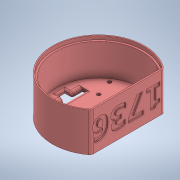
# Autodesk Inventor part: camHolderBottom
Saved by Autodesk Inventor 2020 (Build 240168000, 168)
## iProperties
Created: 2020-02-08
Part Number: camHolderBottom
Material: Generic
Document SubType Name: Modeling
Designer: Chris Gerth
Density: 1 g/cm^3
Appearance: Default(1)
Author: Chris Gerth
Autodesk Inventor part; units mm, degrees
ref_plane "YZ Plane" through (0, 0, 0) normal (1, 0, 0) x (0, 1, 0)
ref_plane "XZ Plane" through (0, 0, 0) normal (0, 1, 0) x (-1, 0, 0)
ref_plane "XY Plane" through (0, 0, 0) normal (0, 0, 1) x (1, 0, 0)
sketch "Sketch1" plane through (0, 0, 0) normal (0, 1, 0) x (-1, 0, 0)
  arc A0 (-25.4, -31.7246) -> (-25.4, 31.7246) centre (0, 0) ccw
  line L0 (-25.4, 31.7246) -> (-25.4, -31.7246)
  dimension "d0" = 81.28
  dimension "d31" = 25.4
  constraints: 2 end point, 2 point on circle, 1 centre point, 1 coincident, 1 vertical
  measures "d0" diameter of A0
  measures "d31" distance from line of L0 point (0, 0)
extrude "Extrusion1" add sketch "Sketch1" along normal blind 3.175
sketch "Sketch2" plane through (0, 3.175, 0) normal (0, 1, 0) x (0, 0, 1)
  arc A0 (-31.7246, 25.4) -> (31.7246, 25.4) centre (0, 0) ccw
  arc A1 (-30.9461, 22.225) -> (30.9461, 22.225) centre (0, 0) ccw
  arc A2 (-31.7246, 25.4) -> (31.7246, 25.4) centre (0, 0) ccw projected
  line L0 (31.7246, 25.4) -> (-31.7246, 25.4)
  line L1 (30.9461, 22.225) -> (-30.9461, 22.225)
  dimension "d3" = 76.2
  dimension "d32" = 3.175
  constraints: 4 end point, 4 point on circle, 2 centre point, 2 coincident, 2 horizontal
  measures "d3" diameter of A1
  measures "d32" distance between parallel lines of L0 L1
extrude "Extrusion2" add sketch "Sketch2" along normal blind 27.94
sketch "Sketch3" plane through (0, 31.115, 0) normal (0, 1, 0) x (0, 0, 1)
  arc A0 (-31.7246, 25.4) -> (31.7246, 25.4) centre (0, 0) ccw
  arc A1 (-31.7246, 25.4) -> (31.7246, 25.4) centre (0, 0) ccw
  arc A2 (-31.5893, 24.13) -> (31.5893, 24.13) centre (0, 0) ccw
  arc A3 (-31.7246, 25.4) -> (31.7246, 25.4) centre (0, 0) ccw projected
  line L0 (31.7246, 25.4) -> (-31.7246, 25.4)
  line L1 (31.5893, 24.13) -> (-31.5893, 24.13)
  dimension "d6" = 79.502
  dimension "d33" = 1.27
  constraints: 6 point on circle, 4 end point, 3 centre point, 3 coincident, 2 horizontal
  measures "d6" diameter of A2
  measures "d33" distance between parallel lines of L0 L1
extrude "Extrusion3" add sketch "Sketch3" along normal blind 3.175
sketch "Sketch4" plane through (0, 3.175, 0) normal (0, 1, 0) x (0, 0, 1)
  line L0 (-14.4, 14.4) -> (14.4, 14.4)
  line L1 (14.4, 14.4) -> (14.4, -14.4)
  line L2 (14.4, -14.4) -> (-14.4, -14.4)
  line L3 (-14.4, -14.4) -> (-14.4, 14.4)
  line L4 (-14.4, 14.4) -> (14.4, -14.4) construction
  line L5 (14.4, 14.4) -> (-14.4, -14.4) construction
  circle A0 centre (-14.4, 14.4) radius 1.55
  circle A1 centre (14.4, 14.4) radius 1.55
  circle A2 centre (-14.4, -14.4) radius 1.55
  circle A3 centre (14.4, -14.4) radius 1.55
  point P0 (0, 0)
  dimension "d9" = 28.8
  dimension "d10" = 28.8
  dimension "d11" = 3.1
  dimension "d12" = 3.1
  dimension "d13" = 3.1
  dimension "d14" = 3.1
  constraints: 12 end point, 4 centre point, 4 coincident, 2 midpoint, 2 parallel, 1 horizontal, 1 perpendicular
  measures "d9" distance of L1.end L2.end
  measures "d10" distance of L2.end L0.start
  measures "d11" diameter of A0
  measures "d12" diameter of A1
  measures "d13" diameter of A2
  measures "d14" diameter of A3
extrude "Extrusion4" cut sketch "Sketch4" against normal up to surface (3.175 mm away) contours L3 A0 L0 | L0 A0 L3 | A1 L1 L0 | L0 L1 A1 | A2 L2 L3 | L3 L2 A2 | A3 L2 L1 | L1 L2 A3
sketch "Sketch5" plane through (0, 3.175, 0) normal (0, 1, 0) x (0, 0, 1)
  line L0 (12.7, -23.7415) -> (-12.7, -23.7415)
  line L1 (-12.7, -23.7415) -> (-12.7, -26.9165)
  line L2 (-12.7, -26.9165) -> (12.7, -26.9165)
  line L3 (12.7, -26.9165) -> (12.7, -23.7415)
  line L4 (12.7, -23.7415) -> (-12.7, -26.9165) construction
  line L5 (-12.7, -23.7415) -> (12.7, -26.9165) construction
  line L6 (3.5906, -33.2771) -> (3.5906, -25.329)
  line L7 (3.5906, -25.329) -> (-3.5906, -25.329)
  line L8 (-3.5906, -25.329) -> (-3.5906, -33.2771)
  line L9 (-3.5906, -33.2771) -> (3.5906, -33.2771)
  line L10 (3.5906, -33.2771) -> (-3.5906, -25.329) construction
  line L11 (3.5906, -25.329) -> (-3.5906, -33.2771) construction
  point P0 (0, 0)
  point P1 (0, -25.329)
  point P2 (0, -29.303)
  point P3 (3.5906, -26.9165)
  point P4 (-3.5906, -26.9165)
  dimension "d17" = 25.4
  dimension "d18" = 3.175
  constraints: 24 end point, 4 midpoint, 4 parallel, 2 perpendicular, 1 vertical
  measures "d17" distance of L0.start L0.end
  measures "d18" distance of L1.end L0.end
extrude "Extrusion5" cut sketch "Sketch5" against normal up to surface (3.175 mm away)
sketch "Sketch6" plane through (0, 3.175, 0) normal (0, 1, 0) x (0, 0, 1)
  line L0 (28.575, 19.05) -> (28.575, -19.05)
  line L1 (28.575, -19.05) -> (-28.575, -19.05)
  line L2 (-28.575, -19.05) -> (-28.575, 19.05)
  line L3 (-28.575, 19.05) -> (28.575, 19.05)
  line L4 (28.575, 19.05) -> (-28.575, -19.05) construction
  line L5 (28.575, -19.05) -> (-28.575, 19.05) construction
  circle A0 centre (-28.575, -19.05) radius 1.55
  circle A1 centre (-28.575, 19.05) radius 1.55
  circle A2 centre (28.575, 19.05) radius 1.55
  circle A3 centre (28.575, -19.05) radius 1.55
  point P0 (0, 0)
  dimension "d21" = 38.1
  dimension "d22" = 57.15
  dimension "d23" = 3.1
  dimension "d24" = 3.1
  dimension "d25" = 3.1
  dimension "d26" = 3.1
  constraints: 12 end point, 4 centre point, 4 coincident, 2 parallel, 1 perpendicular
  measures "d21" distance of L1.end L2.end
  measures "d22" distance of L0.end L1.end
  measures "d23" diameter of A0
  measures "d24" diameter of A1
  measures "d25" diameter of A2
  measures "d26" diameter of A3
extrude "Extrusion6" cut sketch "Sketch6" against normal blind 3.175 contours L3 A2 L0 | L0 A2 L3 | A3 L1 L0 | L0 L1 A3 | A1 L2 L3 | L3 L2 A1 | A0 L2 L1 | L1 L2 A0
sketch "Sketch7" plane through (25.4, 0, 31.7246) normal (1, 0, 0) x (0, 0, -1)
  line L0 (62.4595, 7.7021) -> (-13.7817, 7.7021) construction
  line L1 (-13.7817, 7.7021) -> (-13.7817, 34.1724) construction
  line L2 (-13.7817, 34.1724) -> (62.4595, 34.1724) construction
  line L3 (62.4595, 34.1724) -> (62.4595, 7.7021) construction
  line L4 (48.3825, 25.8567) -> (60.1253, 25.8567)
  line L5 (60.1253, 25.8567) -> (60.1253, 22.7589)
  line L6 (60.1253, 22.7589) -> (56.3791, 22.7589)
  line L7 (56.3791, 22.7589) -> (56.3791, 13.3502)
  line L8 (56.3791, 13.3502) -> (60.1253, 13.3502)
  line L9 (60.1253, 13.3502) -> (60.1253, 10.4541)
  spline S0 degree 2 poles (60.1253, 10.4541) (59.304, 10.4541) (57.6759, 10.2379) (57.186, 10.0074) knots 0 0 0 1 2 2 2
  spline S1 degree 2 poles (57.186, 10.0074) (56.6241, 9.7192) (55.9901, 8.7539) (55.9325, 8.0335) knots 0 0 0 1 2 2 2
  line L10 (55.9325, 8.0335) -> (52.0422, 8.0335)
  line L11 (52.0422, 8.0335) -> (52.0422, 22.7589)
  line L12 (52.0422, 22.7589) -> (48.3825, 22.7589)
  line L13 (48.3825, 22.7589) -> (48.3825, 25.8567)
  line L14 (32.4035, 11.6067) -> (39.9967, 25.8567)
  line L15 (39.9967, 25.8567) -> (44.9532, 25.8567)
  line L16 (44.9532, 25.8567) -> (37.0142, 11.4338)
  line L17 (37.0142, 11.4338) -> (45.4864, 11.4338)
  line L18 (45.4864, 11.4338) -> (45.4864, 8.0767)
  line L19 (45.4864, 8.0767) -> (32.4035, 8.0767)
  line L20 (32.4035, 8.0767) -> (32.4035, 11.6067)
  spline S2 degree 2 poles (16.8856, 20.4679) (16.8856, 21.7791) (17.851, 23.926) (18.7875, 24.6752) knots 0 0 0 1 2 2 2
  spline S3 degree 2 poles (18.7875, 24.6752) (19.7241, 25.4244) (22.2744, 26.2313) (24.1043, 26.2313) knots 0 0 0 1 2 2 2
  spline S4 degree 2 poles (24.1043, 26.2313) (26.1791, 26.2313) (29.1472, 25.5397) (30.0837, 25.1074) knots 0 0 0 1 2 2 2
  line L21 (30.0837, 25.1074) -> (30.0837, 21.246)
  line L22 (30.0837, 21.246) -> (29.6515, 21.246)
  spline S5 degree 2 poles (29.6515, 21.246) (28.6717, 21.8655) (26.035, 22.7877) (24.9399, 22.7877) knots 0 0 0 1 2 2 2
  spline S6 degree 2 poles (24.9399, 22.7877) (24.2916, 22.7877) (22.7787, 22.5572) (22.26, 22.1825) knots 0 0 0 1 2 2 2
  spline S7 degree 2 poles (22.26, 22.1825) (21.8565, 21.88) (21.3666, 21.001) (21.3666, 20.2086) knots 0 0 0 1 2 2 2
  spline S8 degree 2 poles (21.3666, 20.2086) (21.3666, 19.4161) (22.0583, 18.566) (22.6346, 18.3643) knots 0 0 0 1 2 2 2
  spline S9 degree 2 poles (22.6346, 18.3643) (23.2109, 18.1626) (24.8103, 18.1194) (25.4298, 18.1194) knots 0 0 0 1 2 2 2
  line L23 (25.4298, 18.1194) -> (26.1935, 18.1194)
  line L24 (26.1935, 18.1194) -> (26.1935, 14.9927)
  line L25 (26.1935, 14.9927) -> (25.4875, 14.9927)
  spline S10 degree 2 poles (25.4875, 14.9927) (24.6806, 14.9927) (23.3118, 14.8486) (22.8363, 14.6325) knots 0 0 0 1 2 2 2
  spline S11 degree 2 poles (22.8363, 14.6325) (22.3608, 14.402) (21.8277, 13.5951) (21.8277, 12.9035) knots 0 0 0 1 2 2 2
  spline S12 degree 2 poles (21.8277, 12.9035) (21.8277, 12.356) (22.332, 11.6788) (22.6922, 11.4915) knots 0 0 0 1 2 2 2
  spline S13 degree 2 poles (22.6922, 11.4915) (23.1245, 11.2754) (24.2772, 11.1313) (24.6806, 11.1313) knots 0 0 0 1 2 2 2
  spline S14 degree 2 poles (24.6806, 11.1313) (25.329, 11.1313) (26.6978, 11.4338) (27.3317, 11.6788) knots 0 0 0 1 2 2 2
  spline S15 degree 2 poles (27.3317, 11.6788) (27.836, 11.8661) (28.9311, 12.4713) (29.1904, 12.6297) knots 0 0 0 1 2 2 2
  line L26 (29.1904, 12.6297) -> (29.565, 12.6297)
  line L27 (29.565, 12.6297) -> (29.565, 8.8259)
  spline S16 degree 2 poles (29.565, 8.8259) (28.6429, 8.4369) (25.5307, 7.7021) (23.9025, 7.7021) knots 0 0 0 1 2 2 2
  spline S17 degree 2 poles (23.9025, 7.7021) (22.3176, 7.7021) (19.9834, 8.2496) (19.1622, 8.7827) knots 0 0 0 1 2 2 2
  spline S18 degree 2 poles (19.1622, 8.7827) (18.2544, 9.3446) (17.3467, 11.0736) (17.3467, 12.1543) knots 0 0 0 1 2 2 2
  spline S19 degree 2 poles (17.3467, 12.1543) (17.3467, 13.6816) (19.1045, 15.9581) (20.5454, 16.2895) knots 0 0 0 1 2 2 2
  line L28 (20.5454, 16.2895) -> (20.5454, 16.4624)
  spline S20 degree 2 poles (20.5454, 16.4624) (19.9114, 16.5488) (18.7011, 17.0099) (18.1248, 17.5286) knots 0 0 0 1 2 2 2
  spline S21 degree 2 poles (18.1248, 17.5286) (17.5916, 17.9897) (16.8856, 19.4593) (16.8856, 20.4679) knots 0 0 0 1 2 2 2
  spline S22 degree 2 poles (0.9643, 19.8051) (0.9643, 22.6148) (4.5232, 26.2313) (7.6354, 26.2313) knots 0 0 0 1 2 2 2
  spline S23 degree 2 poles (7.6354, 26.2313) (9.1915, 26.2313) (11.6266, 25.338) (12.4766, 24.4591) knots 0 0 0 1 2 2 2
  spline S24 degree 2 poles (12.4766, 24.4591) (13.4852, 23.4361) (14.5659, 20.1942) (14.5659, 17.932) knots 0 0 0 1 2 2 2
  spline S25 degree 2 poles (14.5659, 17.932) (14.5659, 15.5979) (13.5573, 11.967) (12.419, 10.5693) knots 0 0 0 1 2 2 2
  spline S26 degree 2 poles (12.419, 10.5693) (11.3384, 9.2438) (7.8227, 7.7453) (5.4165, 7.7453) knots 0 0 0 1 2 2 2
  spline S27 degree 2 poles (5.4165, 7.7453) (4.5376, 7.7453) (2.7798, 7.9758) (2.4628, 8.0479) knots 0 0 0 1 2 2 2
  line L29 (2.4628, 8.0479) -> (2.4628, 11.5347)
  line L30 (2.4628, 11.5347) -> (2.7798, 11.5347)
  spline S28 degree 2 poles (2.7798, 11.5347) (3.0968, 11.3762) (4.5376, 10.9872) (5.4597, 10.9872) knots 0 0 0 1 2 2 2
  spline S29 degree 2 poles (5.4597, 10.9872) (7.549, 10.9872) (9.8255, 13.1917) (10.0993, 15.2377) knots 0 0 0 1 2 2 2
  spline S30 degree 2 poles (10.0993, 15.2377) (9.2203, 14.6757) (7.4193, 14.013) (6.281, 14.013) knots 0 0 0 1 2 2 2
  spline S31 degree 2 poles (6.281, 14.013) (5.3157, 14.013) (3.6299, 14.5317) (2.9815, 15.0215) knots 0 0 0 1 2 2 2
  spline S32 degree 2 poles (2.9815, 15.0215) (2.0594, 15.7276) (0.9643, 18.0185) (0.9643, 19.8051) knots 0 0 0 1 2 2 2
  spline S33 degree 2 poles (6.1658, 22.4851) (5.82, 22.0529) (5.4453, 21.0443) (5.4453, 20.0213) knots 0 0 0 1 2 2 2
  spline S34 degree 2 poles (5.4453, 20.0213) (5.4453, 19.1568) (5.8776, 18.0329) (6.2666, 17.7015) knots 0 0 0 1 2 2 2
  spline S35 degree 2 poles (6.2666, 17.7015) (6.6701, 17.3557) (7.6642, 17.1108) (8.2262, 17.1108) knots 0 0 0 1 2 2 2
  spline S36 degree 2 poles (8.2262, 17.1108) (8.7016, 17.1108) (9.6814, 17.3557) (10.1137, 17.5286) knots 0 0 0 1 2 2 2
  spline S37 degree 2 poles (10.1137, 17.5286) (10.1137, 17.6439) (10.1425, 18.1914) (10.1425, 18.6092) knots 0 0 0 1 2 2 2
  spline S38 degree 2 poles (10.1425, 18.6092) (10.1425, 20.1509) (9.6094, 22.0096) (9.1915, 22.4851) knots 0 0 0 1 2 2 2
  spline S39 degree 2 poles (9.1915, 22.4851) (8.889, 22.8741) (8.0821, 23.2055) (7.6498, 23.2055) knots 0 0 0 1 2 2 2
  spline S40 degree 2 poles (7.6498, 23.2055) (7.2896, 23.2055) (6.4539, 22.8453) (6.1658, 22.4851) knots 0 0 0 1 2 2 2
  point P0 (31.7246, 0)
  constraints: 2 other
extrude "Extrusion7" cut sketch "Sketch7" against normal blind 1.016
fillet "Fillet1" radius 3.175 2 edges at (25.4, 17.145, 31.7246) (25.4, 17.145, -31.7246)
fillet "Fillet3" radius 3.175 3 edges at (-23.7415, 3.175, 0) (-26.9165, 3.175, -8.1453) (-26.9165, 3.175, 8.1453)
fillet "Fillet4" radius 1.5875 7 edges at (-33.2771, 3.175, 0) (-26.9165, 0.0001, -3.5906) (-27.8464, 2.2451, -3.5906) (-31.6842, 3.175, -3.5906) (-26.9165, 0.0001, 3.5906) (-27.8464, 2.2451, 3.5906) (-31.6842, 3.175, 3.5906)
body "Solid1"
